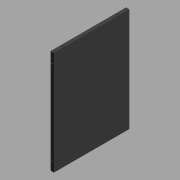
# Autodesk Inventor part: box_side
Saved by Autodesk Inventor 2019 (Build 230136000, 136)
## iProperties
Part Number: box_side
Material: Generic
Document SubType Name: Modeling
Designer: Javi
Appearance: Default
Author: Javi
Autodesk Inventor part; units mm, degrees
ref_plane "YZ Plane" through (0, 0, 0) normal (1, 0, 0) x (0, 1, 0)
ref_plane "XZ Plane" through (0, 0, 0) normal (0, 1, 0) x (-1, 0, 0)
ref_plane "XY Plane" through (0, 0, 0) normal (0, 0, 1) x (1, 0, 0)
sketch "Sketch1" plane through (0, 0, 0) normal (0, 0, 1) x (1, 0, 0)
  line L0 (0, 0) -> (10, 0)
  line L1 (10, 0) -> (10, 310)
  line L2 (10, 310) -> (0, 310)
  line L3 (0, 310) -> (0, 0)
  dimension "d0" = 10
  dimension "d1" = 310
  constraints: 8 end point, 2 parallel, 1 horizontal, 1 perpendicular
  measures "d0" distance of L2.end L1.end
  measures "d1" distance of L1.end L0.end
extrude "Extrusion1" add sketch "Sketch1" along normal blind 226
sketch "Sketch2" plane through (0, 0, 226) normal (0, 0, 1) x (1, 0, 0)
  circle A0 centre (5, 30) radius 2
  line L0 (0, 0) -> (10, 0) projected
  line L1 (0, 310) -> (0, 0) projected
  circle A1 centre (5, 280) radius 2
  dimension "d4" = 4
  dimension "d5" = 30
  dimension "d6" = 5
  dimension "d9" = 250
  constraints: 2 centre point, 1 vertical, 2 other
  measures "d4" diameter of A0
  measures "d5" distance from line of L0 A0.centre
  measures "d6" distance from line of L1 A0.centre
  measures "d9" distance of A0.centre A1.centre
extrude "Extrusion2" cut sketch "Sketch2" against normal blind 20
sketch "Sketch3" plane through (0, 0, 0) normal (0, 0, -1) x (-1, 0, 0)
  circle A0 centre (-5, 30) radius 2
  line L0 (0, 0) -> (-10, 0) projected
  line L1 (-10, 0) -> (-10, 310) projected
  circle A1 centre (-5, 280) radius 2
  dimension "d16" = 4
  dimension "d17" = 30
  dimension "d18" = 5
  dimension "d21" = 250
  constraints: 2 centre point, 1 vertical, 2 other
  measures "d16" diameter of A0
  measures "d17" distance from line of L0 A0.centre
  measures "d18" distance from line of A0.centre L1
  measures "d21" distance of A0.centre A1.centre
extrude "Extrusion3" cut sketch "Sketch3" against normal blind 20
sketch "Sketch4" plane through (0, 0, 0) normal (0, -1, 0) x (1, 0, 0)
  circle A0 centre (5, 30) radius 2
  line L0 (0, 0) -> (10, 0) projected
  line L1 (0, 0) -> (0, 226) projected
  circle A1 centre (5, 196) radius 2
  dimension "d28" = 4
  dimension "d29" = 30
  dimension "d30" = 5
  dimension "d33" = 166
  constraints: 2 centre point, 1 vertical, 2 other
  measures "d28" diameter of A0
  measures "d29" distance from line of L0 A0.centre
  measures "d30" distance from line of L1 A0.centre
  measures "d33" distance of A0.centre A1.centre
extrude "Extrusion4" cut sketch "Sketch4" against normal blind 20
sketch "Sketch5" plane through (10, 0, 0) normal (1, 0, 0) x (0, 0, -1)
  circle A0 centre (-196, 205) radius 2
  line L0 (0, 0) -> (-226, 0) projected
  line L1 (-226, 0) -> (-226, 310) projected
  circle A1 centre (-20, 205) radius 2
  dimension "d40" = 4
  dimension "d41" = 205
  dimension "d42" = 30
  dimension "d45" = 176
  constraints: 2 centre point, 1 horizontal, 2 other
  measures "d40" diameter of A0
  measures "d41" distance from line of L0 A0.centre
  measures "d42" distance from line of L1 A0.centre
  measures "d45" distance of A0.centre A1.centre
extrude "Extrusion5" cut sketch "Sketch5" against normal through all
sketch "Sketch6" plane through (0, 310, 0) normal (0, 1, 0) x (1, 0, 0)
  circle A0 centre (5, -30) radius 2
  line L0 (10, 0) -> (10, -226) projected
  line L1 (10, 0) -> (0, 0) projected
  circle A1 centre (5, -196) radius 2
  dimension "d52" = 4
  dimension "d53" = 5
  dimension "d54" = 30
  dimension "d57" = 166
  constraints: 2 centre point, 1 vertical, 2 other
  measures "d52" diameter of A0
  measures "d53" distance from line of L0 A0.centre
  measures "d54" distance from line of L1 A0.centre
  measures "d57" distance of A0.centre A1.centre
extrude "Extrusion6" cut sketch "Sketch6" against normal blind 20
equation "\"d40\" = screws"
equation "\"d52\" = screws"
equation "\"screws\" = 4"
body "Solid1"
